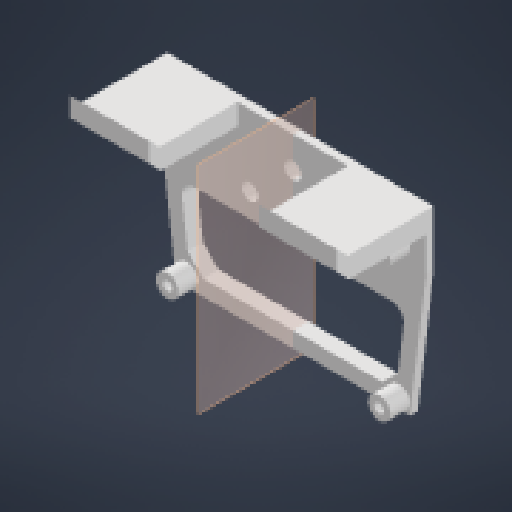
# Autodesk Inventor part: Esp32_Holder
Saved by Autodesk Inventor 2024 (Build 280153000, 153)
## iProperties
Created: 2025-10-03
Part Number: Esp32_Holder
Material: Generic
Document SubType Name: Modeling
Designer: kevin
Density: 1 g/cm^3
Appearance: Default
Author: kevin
Autodesk Inventor part; units mm, degrees
ref_plane "XZ Plane" through (0, 0, 0) normal (0, 1, 0) x (-1, 0, 0)
ref_plane "XY Plane" through (0, 0, 0) normal (0, 0, 1) x (1, 0, 0)
sketch "Sketch1" plane through (0, 0, 0) normal (0, 0, 1) x (1, 0, 0)
  circle A0 centre (0, 35.5533) radius 2.1 projected
  circle A1 centre (11, 25.3552) radius 2.1 projected
  circle A2 centre (-11, 25.3552) radius 2.1 projected
  circle A3 centre (6.25, -60.9016) radius 2.1 projected
  circle A4 centre (-33.6286, -15.6738) radius 2.1 projected
  circle A5 centre (-5.75, -60.9016) radius 2.1 projected
  circle A6 centre (34.1286, -15.6738) radius 2.1 projected
  circle A7 centre (-24.1373, -40.1344) radius 6.75 projected
  circle A8 centre (24.6373, -40.1344) radius 6.75 projected
  circle A9 centre (10.7484, -21.5639) radius 2.1 projected
  circle A10 centre (-10.2484, -21.5639) radius 2.1 projected
  line L0 (-59, -41.44) -> (-59, -14.3421) projected
  line L1 (-59, -41.44) -> (-53, -41.44) projected
  line L2 (-53, -41.44) -> (-53, -91.44) projected
  line L3 (-53, -91.44) -> (53, -91.44) projected
  line L4 (53, -91.44) -> (53, -41.44) projected
  line L5 (53, -41.44) -> (59, -41.44) projected
  line L6 (59, -14.3421) -> (59, -41.44) projected
  line L7 (59, -14.3421) -> (54, -14.3421) projected
  line L8 (54, -14.3421) -> (54, 35.0192) projected
  line L9 (54, 35.0192) -> (59, 35.0192) projected
  line L10 (59, 80.19) -> (59, 35.0192) projected
  line L11 (59, 80.19) -> (46.35, 80.19) projected
  line L12 (46.35, 80.19) -> (46.35, 63.44) projected
  line L13 (46.35, 63.44) -> (-46.35, 63.44) projected
  line L14 (-46.35, 63.44) -> (-46.35, 80.19) projected
  line L15 (-46.35, 80.19) -> (-59, 80.19) projected
  line L16 (-59, 35.0192) -> (-59, 80.19) projected
  line L17 (-59, 35.0192) -> (-54, 35.0192) projected
  line L18 (-54, 35.0192) -> (-54, -14.3421) projected
  line L19 (-54, -14.3421) -> (-59, -14.3421) projected
  circle A11 centre (0, 35.5533) radius 6.1 construction
  line L20 (34.1312, 49.9126) -> (34.1312, 18.1374) construction
  line L21 (-34.1313, 18.1374) -> (-34.1313, 49.9126) construction
  line L22 (34.1312, 43.6533) -> (-34.1313, 43.6533)
  line L23 (-34.1313, 43.6533) -> (-34.1312, 29.7711)
  line L24 (-30.0745, -3.9522) -> (30.0745, -3.9522)
  line L25 (34.1312, 29.7711) -> (34.1312, 43.6533)
  line L26 (-30, -3.9121) -> (30, -3.9121) construction
  line L27 (30, -3.9121) -> (30, 36.0879) construction
  line L28 (30, 36.0879) -> (-30, 36.0879) construction
  line L29 (-30, 36.0879) -> (-30, -3.9121) construction
  line L30 (-30, -3.9121) -> (30, 36.0879) construction
  line L31 (30, -3.9121) -> (-30, 36.0879) construction
  line L32 (-34.1312, 29.7711) -> (-30.0745, -3.9522)
  line L33 (0, 16.0879) -> (0, 8.3045) construction
  line L34 (34.1312, 29.7711) -> (30.0745, -3.9522)
  line L35 (26.5268, 0.0478) -> (-26.5268, 0.0478)
  line L36 (-26.5268, 0.0478) -> (-30.1312, 30.0109)
  line L37 (-30.1312, 30.0109) -> (-30.1312, 39.6533)
  line L38 (-30.1312, 39.6533) -> (30.1312, 39.6533)
  line L39 (30.1312, 39.6533) -> (30.1312, 30.0109)
  line L40 (30.1312, 30.0109) -> (26.5268, 0.0478)
  line L41 (-28.8342, 19.2288) -> (28.8342, 19.2288)
  line L42 (-27.0103, 4.0668) -> (-22.9193, 0.0478)
  line L43 (27.0103, 4.0668) -> (22.9193, 0.0478)
  point P0 (0, 0)
  point P1 (30.0601, -3.9522)
  point P2 (34.1312, 29.891)
  point P3 (22.9193, 0.0478)
  dimension "d0" = 4
  dimension "d3" = 60
  dimension "d4" = 40
  dimension "d5" = 4
  constraints: 44 end point, 7 parallel, 5 point on line, 4 symmetric about line, 3 perpendicular, 2 horizontal, 2 midpoint, 1 centre point, 1 vertical, 5 other
  measures "d0" radial gap between concentric circles of A0 A11
  measures "d3" distance of L28.end L27.end
  measures "d4" distance of L27.end L26.end
  measures "d5" distance between parallel lines of L24 L35
extrude "Extrusion1" add sketch "Sketch1" along normal blind 4 contours L25 L34 L24 L32 L23 L22 | L35 L43 L40 | L35 L36 L42 | L41 L36 L37 L38 L39 L40
sketch "Sketch2" plane through (0, 0, 4) normal (0, 0, 1) x (1, 0, 0)
  line L0 (-30, 36.0478) -> (30, 36.0478)
  line L1 (30, 36.0478) -> (30, -3.9522)
  line L2 (30, -3.9522) -> (-30, -3.9522)
  line L3 (-30, -3.9522) -> (-30, 36.0478)
  line L4 (-30, 36.0478) -> (30, -3.9522) construction
  line L5 (30, 36.0478) -> (-30, -3.9522) construction
  line L6 (-30.0745, -3.9522) -> (30.0745, -3.9522) construction
  circle A0 centre (27.15, -1.1022) radius 1 construction
  circle A1 centre (27.15, -1.1022) radius 1.2
  circle A2 centre (27.15, -1.1022) radius 2.85
  line L7 (30, 16.0478) -> (-30, 16.0478) construction
  line L8 (0, 36.0478) -> (0, -3.9522) construction
  circle A3 centre (27.15, 33.1978) radius 1.2
  circle A4 centre (27.15, 33.1978) radius 2.85
  circle A5 centre (-27.15, -1.1022) radius 1.2
  circle A6 centre (-27.15, -1.1022) radius 2.85
  circle A7 centre (-27.15, 33.1978) radius 1.2
  circle A8 centre (-27.15, 33.1978) radius 2.85
  point P0 (0, 0)
  point P1 (0, 16.0478)
  dimension "d6" = 60
  dimension "d7" = 40
  dimension "d8" = 2
  dimension "d9" = 2.85
  dimension "d10" = 2.85
  dimension "d11" = 0.2
  constraints: 16 end point, 9 centre point, 6 midpoint, 3 symmetric about line, 2 parallel, 1 horizontal, 1 perpendicular, 1 point on line, 1 tangent, 6 other
  measures "d6" distance of L1.end L2.end
  measures "d7" distance of L0.end L1.end
  measures "d8" diameter of A0
  measures "d9" distance from line of L1 A0.centre
  measures "d10" distance from line of L2 A0.centre
  measures "d11" radial gap between concentric circles of A0 A1
extrude "Extrusion2" add sketch "Sketch2" along normal blind 5 contours A8 | A4 | A6 | A2
sketch "Sketch3" plane through (-34.1312, 29.7711, 0) normal (-1, 0, 0) x (0, 0, 1)
  line L0 (4, 13.8821) -> (4, 0) projected
  line L1 (4, 13.8821) -> (24, 13.8821)
  line L2 (24, 13.8821) -> (24, 8.5067)
  line L3 (24, 8.5067) -> (4, 8.5067)
  line L4 (4, 8.5067) -> (4, 13.8821)
  line L5 (24, 13.8821) -> (26.8284, 16.7106)
  line L6 (24, 13.8821) -> (28, 13.8821) construction
  line L7 (26.8284, 16.7106) -> (26.8284, 8.5067)
  line L8 (26.8284, 8.5067) -> (24, 8.5067)
  point P0 (0, -29.7711)
  point P1 (4, 8.5067)
  dimension "d14" = 20
  dimension "d15" = 4
  dimension "d16" = 45
  constraints: 16 end point, 2 horizontal, 2 parallel, 2 perpendicular, 1 equal length, 1 vertical
  measures "d14" distance of L2.end L3.end
  measures "d15" distance of L1.end L5.end
  measures "d16" angle of L6 L5
extrude "Extrusion3" add sketch "Sketch3" against normal blind 20
chamfer "Chamfer1" distance 3.175 angle 45 1 edges at (-24.1313, 38.2779, 26.8284)
chamfer "Chamfer2" distance 2 angle 45 6 edges at (-32.1029, 12.9095, 0) (0, -3.9522, 0) (32.1029, 12.9095, 0) (34.1312, 36.7122, 0) (0, 43.6533, 0) (-34.1313, 36.7122, 0)
fillet "Fillet1" radius 3.175 2 edges at (28.8342, 19.2288, 2) (-28.8342, 19.2288, 2)
mirror "Mirror1" about plane through (0, 0, 0) normal (1, 0, 0) of "Extrusion3", "Chamfer1"
equation "\"d10\" = d9"
body "Solid1"
